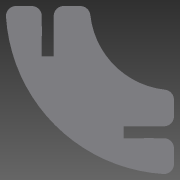
# Autodesk Inventor part: circle
Saved by Autodesk Inventor 2015 (Build 190159000, 159)
## iProperties
Created: 2015-02-16
Part Number: circle
Material: Generic
Document SubType Name: Modeling
Designer: Iain
Density: 1 g/cm^3
Appearance: Default
Author: Iain
Autodesk Inventor part; units mm, degrees
ref_plane "YZ Plane" through (0, 0, 0) normal (1, 0, 0) x (0, 1, 0)
derived "hex.ipt"
sketch "Sketch1" plane through (0, 0, 0) normal (0, 1, 0) x (-1, 0, 0)
  circle A0 centre (0, 0) radius 25 construction
  circle A1 centre (0, 0) radius 33.3333
  circle A2 centre (0, 0) radius 16.6667
  line L0 (0, 0) -> (-40.392, 44.0905) construction
  dimension "d1" = 25
  dimension "d2" = 8.3333
  dimension "d3" = 8.3333
  constraints: 3 centre point, 3 coincident, 2 end point
  measures "d1" radius of A0
  measures "d2" radial gap between concentric circles of A1 A0
  measures "d3" radial gap between concentric circles of A0 A2
extrude "Extrusion1" add sketch "Sketch1" along normal blind 2.5
sketch "Sketch2" plane through (0, 2.5, 0) normal (0, 1, 0) x (1, 0, 0)
  circle A0 centre (0, 0) radius 16.6667 projected
  circle A1 centre (0, 0) radius 33.3333 projected
  line L0 (-33.3333, -33.3333) -> (0, -33.3333)
  line L1 (0, -33.3333) -> (0, 0)
  line L2 (0, 0) -> (-33.3333, 0)
  line L3 (-33.3333, 0) -> (-33.3333, -33.3333)
  constraints: 8 end point, 2 parallel, 2 point on circle, 1 coincident, 1 horizontal, 1 perpendicular
extrude "Extrusion2" cut sketch "Sketch2" against normal through all contours L2 L1 A0 | A0 L1 A1 L2 keep common part picked at (-10.9718, -1.2362) picked at (-27.4992, -2.4725)
sketch "Sketch3" plane through (0, 2.5, 0) normal (0, 1, 0) x (1, 0, 0)
  line L0 (0, -16.6667) -> (0, -33.3333) projected
  line L1 (-10, -26.175) -> (0, -26.175)
  line L2 (0, -26.175) -> (0, -23.825)
  line L3 (0, -23.825) -> (-10, -23.825)
  line L4 (-10, -23.825) -> (-10, -26.175)
  point P0 (0, -25)
  point P1 (0, -25)
  point P2 (0, -25)
  dimension "d8" = 2.35
  dimension "d9" = 10
  constraints: 8 end point, 3 midpoint, 2 coincident, 2 parallel, 1 horizontal, 1 perpendicular
  measures "d8" distance of L3.end L1.start
  measures "d9" distance of L2.end L3.end
extrude "Extrusion3" cut sketch "Sketch3" against normal blind 2.5
sketch "Sketch4" plane through (0, 2.5, 0) normal (0, 1, 0) x (1, 0, 0)
  line L0 (-10, -23.825) -> (0, -23.825) projected
  arc A0 (-6.25, -23.825) -> (-3.75, -23.825) centre (-5, 7.4125) ccw
  line L1 (-14.7231, -23.85) -> (1.6524, -23.85) construction
  line L2 (-6.25, -23.825) -> (-3.75, -23.825)
  point P0 (-5, -23.825)
  point P1 (-5, -23.825)
  point P2 (-5, -23.825)
  dimension "d12" = 2.5
  dimension "d13" = 0.025
  constraints: 4 end point, 3 midpoint, 2 horizontal alignment, 2 point on circle, 1 centre point, 1 horizontal, 1 tangent, 1 vertical alignment
  measures "d12" distance of L2.end L2.start
  measures "d13" distance from line of L1 point (-5, -23.825)
extrude "Extrusion4" add sketch "Sketch4" against normal blind 2.5
ref_plane "Work Plane1" through (-10, 0, 25) normal (0, 0, 1) x (1, 0, 0)
mirror "Mirror1" about plane through (-10, 0, 25) normal (0, 0, 1) of "Extrusion4"
ref_plane "Work Plane2" through (0, 2.5, 0) normal (-0.7071068, 0, -0.7071068) x (0, 1, 0)
mirror "Mirror2" about plane through (0, 2.5, 0) normal (-0.7071068, 0, -0.7071068) of "Extrusion3", "Extrusion4", "Mirror1"
fillet "slotFillet" radius 2 4 edges at (-26.175, 1.25, 0) (-23.825, 1.25, 0) (0, 1.25, 23.825) (0, 1.25, 26.175)
fillet "edgeFillet" radius 2 4 edges at (-33.3333, 1.25, 0) (-16.6667, 1.25, 0) (0, 1.25, 33.3333) (0, 1.25, 16.6667)
equation "\"d1\" = 0.5 * hexWidth"
equation "\"d2\" = 0.166667 * hexWidth"
equation "\"d3\" = d2"
equation "\"d4\" = materialThickness"
equation "\"d6\" = materialThickness"
equation "\"d8\" = slotWidth"
equation "\"d9\" = slotDepth"
equation "\"d10\" = materialThickness"
equation "\"d12\" = 0.25 * slotDepth"
equation "\"d13\" = slotNoduleHeight"
equation "\"d14\" = materialThickness"
equation "\"hexWidth\" = 50"
equation "\"materialThickness\" = 2.5"
equation "\"slotWidth\" = 2.35"
equation "\"slotDepth\" = 10"
equation "\"slotNoduleHeight\" = 0.025"
body "Solid1"
